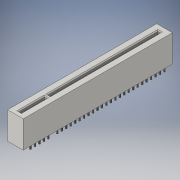
# Autodesk Inventor part: PCI_TH
Saved by Autodesk Inventor 2016 (Build 200138000, 138)
## iProperties
Created: 2017-03-03
Part Number: PCI_TH
Material: Generic
Document SubType Name: Modeling
Designer: jfixelle
Density: 1 g/cm^3
Appearance: White
Author: jfixelle
Autodesk Inventor part; units mm, degrees
note: some values were not read from the file. Chosen so that the rebuilt part matches the saved one: sketch regions of "Extrusion2".
ref_plane "YZ Plane" through (0, 0, 0) normal (1, 0, 0) x (0, 1, 0)
ref_plane "XZ Plane" through (0, 0, 0) normal (0, 1, 0) x (-1, 0, 0)
ref_plane "XY Plane" through (0, 0, 0) normal (0, 0, 1) x (1, 0, 0)
sketch "Sketch1" plane through (0, 0, 0) normal (0, 1, 0) x (-1, 0, 0)
  line L0 (4.445, 18.07) -> (-4.445, 18.07)
  line L1 (-4.445, 18.07) -> (-4.445, -66.77)
  line L2 (-4.445, -66.77) -> (4.445, -66.77)
  line L3 (4.445, -66.77) -> (4.445, 18.07)
  point P0 (0, 0)
  dimension "d0" = 8.89
  dimension "d1" = 4.445
  dimension "d2" = 66.77
  dimension "d3" = 84.84
  constraints: 8 end point, 2 parallel, 1 horizontal, 1 perpendicular
  measures "d0" distance of L1.end L2.end
  measures "d1" distance from line of point (0, 0) L3
  measures "d2" distance from line of L2 point (0, 0)
  measures "d3" distance of L0.end L1.end
extrude "Extrusion1" add sketch "Sketch1" along normal blind 15.49
sketch "Sketch2" plane through (0, 15.49, 0) normal (0, 1, 0) x (1, 0, 0)
  line L0 (-0.8, -15.49) -> (0.8, -15.49)
  line L1 (0.8, -15.49) -> (0.8, 63.76)
  line L2 (0.8, 63.76) -> (-0.8, 63.76)
  line L3 (-0.8, 63.76) -> (-0.8, -15.49)
  line L4 (-0.8, -0.955) -> (0.8, -0.955)
  line L5 (0.8, -0.955) -> (0.8, 0.955)
  line L6 (0.8, 0.955) -> (-0.8, 0.955)
  line L7 (-0.8, 0.955) -> (-0.8, -0.955)
  point P0 (0, 0)
  dimension "d6" = 1.6
  dimension "d7" = 0.8
  dimension "d8" = 15.49
  dimension "d9" = 63.76
  dimension "d10" = 0.955
  dimension "d11" = 1.91
  constraints: 16 end point, 4 parallel, 2 horizontal, 2 perpendicular, 2 point on line
  measures "d6" distance of L1.end L2.end
  measures "d7" distance from line of point (0, 0) L3
  measures "d8" distance from line of L0 point (0, 0)
  measures "d9" distance from line of point (0, 0) L2
  measures "d10" distance from line of point (0, 0) L4
  measures "d11" distance between parallel lines of L6 L4
extrude "Extrusion2" cut sketch "Sketch2" against normal blind 7.87 contours L3 L4 L1 L0 | L3 L2 L1 L6
sketch "Sketch3" plane through (0, 0, 0) normal (0, -1, 0) x (1, 0, 0)
  circle A0 centre (0, 0) radius 1.2
  circle A1 centre (0, -64.77) radius 1.2
  dimension "d14" = 64.77
  dimension "d15" = 2.4
  dimension "d16" = 2.4
  dimension "d17" = 0
  constraints: 2 centre point, 1 coincident
  measures "d14" distance of point (0, 0) A1.centre
  measures "d15" diameter of A1
  measures "d16" diameter of A0
  measures "d17" horizontal distance of point (0, 0) A1.centre
extrude "Extrusion3" add sketch "Sketch3" along normal blind 3
sketch "Sketch4" plane through (0, 0, 0) normal (0, -1, 0) x (1, 0, 0)
  line L0 (-1.27, 14.1621) -> (-1.27, -63.3054) construction
  line L1 (-3.81, 14.1621) -> (-3.81, -66.1848) construction
  circle A0 centre (-1.27, -1.91) radius 0.45
  circle A1 centre (-3.81, -3.18) radius 0.45
  circle A2 centre (-1.27, 3.18) radius 0.45
  circle A3 centre (-3.81, 1.91) radius 0.45
  circle A4 centre (-1.27, -4.45) radius 0.45
  circle A5 centre (-1.27, -6.99) radius 0.45
  circle A6 centre (-1.27, -9.53) radius 0.45
  circle A7 centre (-1.27, -12.07) radius 0.45
  circle A8 centre (-1.27, -14.61) radius 0.45
  circle A9 centre (-1.27, -17.15) radius 0.45
  circle A10 centre (-1.27, -19.69) radius 0.45
  circle A11 centre (-1.27, -22.23) radius 0.45
  circle A12 centre (-1.27, -24.77) radius 0.45
  circle A13 centre (-1.27, -27.31) radius 0.45
  circle A14 centre (-1.27, -29.85) radius 0.45
  circle A15 centre (-1.27, -32.39) radius 0.45
  circle A16 centre (-1.27, -34.93) radius 0.45
  circle A17 centre (-1.27, -37.47) radius 0.45
  circle A18 centre (-1.27, -40.01) radius 0.45
  circle A19 centre (-1.27, -42.55) radius 0.45
  circle A20 centre (-1.27, -45.09) radius 0.45
  circle A21 centre (-1.27, -47.63) radius 0.45
  circle A22 centre (-1.27, -50.17) radius 0.45
  circle A23 centre (-1.27, -52.71) radius 0.45
  circle A24 centre (-1.27, -55.25) radius 0.45
  circle A25 centre (-1.27, -57.79) radius 0.45
  circle A26 centre (-1.27, -60.33) radius 0.45
  circle A27 centre (-1.27, -62.87) radius 0.45
  circle A28 centre (-3.81, -5.72) radius 0.45
  circle A29 centre (-3.81, -8.26) radius 0.45
  circle A30 centre (-3.81, -10.8) radius 0.45
  circle A31 centre (-3.81, -13.34) radius 0.45
  circle A32 centre (-3.81, -15.88) radius 0.45
  circle A33 centre (-3.81, -18.42) radius 0.45
  circle A34 centre (-3.81, -20.96) radius 0.45
  circle A35 centre (-3.81, -23.5) radius 0.45
  circle A36 centre (-3.81, -26.04) radius 0.45
  circle A37 centre (-3.81, -28.58) radius 0.45
  circle A38 centre (-3.81, -31.12) radius 0.45
  circle A39 centre (-3.81, -33.66) radius 0.45
  circle A40 centre (-3.81, -36.2) radius 0.45
  circle A41 centre (-3.81, -38.74) radius 0.45
  circle A42 centre (-3.81, -41.28) radius 0.45
  circle A43 centre (-3.81, -43.82) radius 0.45
  circle A44 centre (-3.81, -46.36) radius 0.45
  circle A45 centre (-3.81, -48.9) radius 0.45
  circle A46 centre (-3.81, -51.44) radius 0.45
  circle A47 centre (-3.81, -53.98) radius 0.45
  circle A48 centre (-3.81, -56.52) radius 0.45
  circle A49 centre (-3.81, -59.06) radius 0.45
  circle A50 centre (-3.81, -61.6) radius 0.45
  circle A51 centre (-3.81, 4.45) radius 0.45
  circle A52 centre (-3.81, 6.99) radius 0.45
  circle A53 centre (-3.81, 9.53) radius 0.45
  circle A54 centre (-3.81, 12.07) radius 0.45
  circle A55 centre (-3.81, 14.61) radius 0.45
  circle A56 centre (-1.27, 5.72) radius 0.45
  circle A57 centre (-1.27, 8.26) radius 0.45
  circle A58 centre (-1.27, 10.8) radius 0.45
  circle A59 centre (-1.27, 13.34) radius 0.45
  line L2 (0, 0) -> (-2.8416, 0)
  circle A60 centre (3.81, -24.77) radius 0.45
  circle A61 centre (1.27, -26.04) radius 0.45
  circle A62 centre (3.81, -27.31) radius 0.45
  circle A63 centre (1.27, -28.58) radius 0.45
  circle A64 centre (3.81, -29.85) radius 0.45
  circle A65 centre (1.27, -31.12) radius 0.45
  circle A66 centre (3.81, -32.39) radius 0.45
  circle A67 centre (3.81, -34.93) radius 0.45
  circle A68 centre (1.27, -36.2) radius 0.45
  circle A69 centre (3.81, -37.47) radius 0.45
  circle A70 centre (1.27, -38.74) radius 0.45
  circle A71 centre (3.81, -40.01) radius 0.45
  circle A72 centre (1.27, -41.28) radius 0.45
  circle A73 centre (1.27, -33.66) radius 0.45
  line L3 (1.27, 14.1621) -> (1.27, -66.1848) construction
  line L4 (3.81, 14.1621) -> (3.81, -63.3054) construction
  circle A74 centre (3.81, -14.61) radius 0.45
  circle A75 centre (1.27, -15.88) radius 0.45
  circle A76 centre (3.81, -17.15) radius 0.45
  circle A77 centre (1.27, -18.42) radius 0.45
  circle A78 centre (3.81, -19.69) radius 0.45
  circle A79 centre (1.27, -20.96) radius 0.45
  circle A80 centre (3.81, -22.23) radius 0.45
  circle A81 centre (1.27, -23.5) radius 0.45
  circle A82 centre (3.81, -1.91) radius 0.45
  circle A83 centre (1.27, -13.34) radius 0.45
  circle A84 centre (3.81, -12.07) radius 0.45
  circle A85 centre (1.27, -10.8) radius 0.45
  circle A86 centre (3.81, -9.53) radius 0.45
  circle A87 centre (3.81, -6.99) radius 0.45
  circle A88 centre (1.27, -5.72) radius 0.45
  circle A89 centre (3.81, -4.45) radius 0.45
  circle A90 centre (1.27, -3.18) radius 0.45
  circle A91 centre (1.27, -8.26) radius 0.45
  circle A92 centre (3.81, -42.55) radius 0.45
  circle A93 centre (3.81, -55.25) radius 0.45
  circle A94 centre (1.27, -53.98) radius 0.45
  circle A95 centre (3.81, -52.71) radius 0.45
  circle A96 centre (1.27, -51.44) radius 0.45
  circle A97 centre (3.81, -50.17) radius 0.45
  circle A98 centre (1.27, -48.9) radius 0.45
  circle A99 centre (3.81, -47.63) radius 0.45
  circle A100 centre (1.27, -46.36) radius 0.45
  circle A101 centre (3.81, -45.09) radius 0.45
  circle A102 centre (1.27, -43.82) radius 0.45
  circle A103 centre (3.81, -57.79) radius 0.45
  circle A104 centre (1.27, -59.06) radius 0.45
  circle A105 centre (3.81, -60.33) radius 0.45
  circle A106 centre (1.27, -61.6) radius 0.45
  circle A107 centre (3.81, -62.87) radius 0.45
  circle A108 centre (1.27, -56.52) radius 0.45
  circle A109 centre (3.81, 3.18) radius 0.45
  circle A110 centre (1.27, 1.91) radius 0.45
  circle A111 centre (1.27, 4.45) radius 0.45
  circle A112 centre (1.27, 6.99) radius 0.45
  circle A113 centre (3.81, 8.26) radius 0.45
  circle A114 centre (1.27, 9.53) radius 0.45
  circle A115 centre (3.81, 10.8) radius 0.45
  circle A116 centre (1.27, 12.07) radius 0.45
  circle A117 centre (3.81, 13.34) radius 0.45
  circle A118 centre (1.27, 14.61) radius 0.45
  circle A119 centre (3.81, 5.72) radius 0.45
  dimension "d20" = 1.27
  dimension "d21" = 3.81
  dimension "d22" = 1.91
  dimension "d23" = 1.27
  dimension "d24" = 0.9
  dimension "d25" = 0.9
  dimension "d26" = 0.9
  dimension "d27" = 0.9
  dimension "d28" = 1.91
  dimension "d29" = 1.27
  dimension "d32" = 2.54
  dimension "d39" = 2.54
  dimension "d46" = 2.54
  dimension "d53" = 2.54
  dimension "d60" = 5.08
  constraints: 120 centre point, 10 end point, 8 point on line, 6 vertical, 2 horizontal, 238 other
  measures "d20" distance from line of L0 L2.start
  measures "d21" distance from line of L1 L2.start
  measures "d22" vertical distance of L2.start A0.centre
  measures "d23" vertical distance of A1.centre A0.centre
  measures "d24" diameter of A0
  measures "d25" diameter of A1
  measures "d26" diameter of A2
  measures "d27" diameter of A3
  measures "d28" vertical distance of L2.start A3.centre
  measures "d29" vertical distance of A3.centre A2.centre
  measures "d32" distance of A0.centre A4.centre
  measures "d39" distance of A1.centre A28.centre
  measures "d46" distance of A3.centre A51.centre
  measures "d53" distance of A2.centre A56.centre
  measures "d60" distance of A12.centre A60.centre
extrude "Extrusion4" add sketch "Sketch4" along normal blind 2
chamfer "Chamfer1" distance 0.5 angle 45 1 edges at (-1.2, -3, -64.77)
chamfer "Chamfer2" distance 0.5 angle 45 1 edges at (-1.2, -3, 0)
chamfer "Chamfer3" distance 0.5 angle 45 4 edges at (0, 15.49, 15.49) (0.8, 15.49, 8.2225) (0, 15.49, 0.955) (-0.8, 15.49, 8.2225)
chamfer "Chamfer4" distance 0.5 angle 45 4 edges at (0, 15.49, -0.955) (-0.8, 15.49, -32.3575) (0.8, 15.49, -32.3575) (0, 15.49, -63.76)
body "Solid1"
